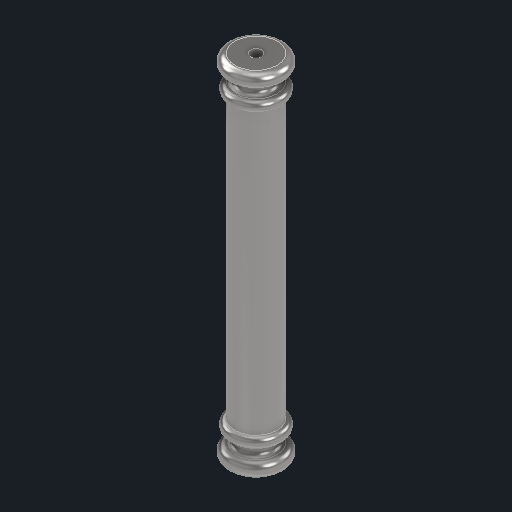
# Autodesk Inventor part: Bell Support Piller
Saved by Autodesk Inventor 2027.1 (Build 311270010, 270A)
## iProperties
Created: 2025-09-17
Material: Stainless Steel
Document SubType Name: Modeling
Designer: SD
Density: 8 g/cm^3
Appearance: Semi-Polished
Mass: 92.5719 g
Surface Area: 49.3716 cm^2
Volume: 11.5715 cm^3
Project: Automatic Tea Steeping mechanism
Part Number: Bell Support Piller
BOM-Mass: 0.09801
BOM-Area: 0.005
DateTimeString: 27-10-25 16:18
Date: 2025-10-27
Length: 100.000 mm
Diameter: 16.000 mm
Procurement: Fabricate - 2nd round
Build Stage: 3
Preferred Material: 303 Stainless Steel
Author: SD
Title: Bell Support Piller
Autodesk Inventor part; units mm, degrees
ref_plane "XZ Plane" through (0, 0, 0) normal (0, 1, 0) x (-1, 0, 0)
ref_plane "XY Plane" through (0, 0, 0) normal (0, 0, 1) x (1, 0, 0)
sketch "Sketch1" plane through (0, 0, 0) normal (0, 0, 1) x (1, 0, 0)
  line L0 (0, 0) -> (0, -100)
  line L1 (0, 0) -> (6, 0)
  line L2 (6, 0) -> (6, -4) construction
  arc A0 (6, -4) -> (6, 0) centre (6, -2) ccw
  arc A1 (6, -4) -> (6, -7) centre (6, -5.5) ccw
  line L3 (6, -5.5) -> (2.7369, -5.5) construction
  arc A2 (6, -10) -> (6, -7) centre (6, -8.5) ccw
  line L4 (0, -100) -> (6, -100)
  line L5 (6, -100) -> (6, -96) construction
  arc A3 (6, -100) -> (6, -96) centre (6, -98) ccw
  arc A4 (6, -93) -> (6, -96) centre (6, -94.5) ccw
  arc A5 (6, -93) -> (6, -90) centre (6, -91.5) ccw
  line L6 (6, -10) -> (6, -90)
  point P0 (6, -90)
  point P1 (6, -10)
  dimension "d1" = 8
  dimension "d2" = 4
  dimension "d3" = 1.5
  dimension "d4" = 3
  dimension "d5" = 3
  dimension "d6" = 1.5
  dimension "d7" = 4
  dimension "d8" = 8
  dimension "d9" = 1.5
  dimension "d10" = 3
  dimension "d11" = 3
  dimension "d12" = 1.5
  dimension "d47" = 80
  constraints: 14 end point, 12 point on circle, 6 centre point, 5 vertical alignment, 4 vertical, 3 horizontal, 2 midpoint
  measures "d2" distance of L1.end L2.end
  measures "d3" radius of A1
  measures "d4" distance of A1.end L2.end
  measures "d5" distance of A1.end L6.start
  measures "d6" radius of A2
  measures "d7" distance of L4.end L5.end
  measures "d9" radius of A4
  measures "d10" distance of L5.end A4.start
  measures "d11" distance of A4.start A5.end
  measures "d12" radius of A5
  measures "d47" distance of L6.start L6.end
revolve "Revolution1" add sketch "Sketch1" angle 360 about axis through (0, 0, 0) along (0, -1, 0)
ref_plane "Work Plane1" through (8, 0, 0) normal (1, 0, 0) x (0, 1, 0)
ref_plane "Work Plane2" through (-8, 0, 0) normal (1, 0, 0) x (0, 1, 0)
sketch "Sketch5" plane through (0, -100, 0) normal (0, -1, 0) x (1, 0, 0)
  point P0 (0, 0)
  point P1 (0, 0)
  constraints: 1 coincident
hole "Hole1" at (0, -100, 0) direction (0, 1, 0) diameter 3.242 depth 20 tip angle 118 thread size "M4x0.7" class "6H" standard "ISO Metric profile"
sketch "Sketch6" plane through (0, 0, 0) normal (0, 1, 0) x (1, 0, 0)
  point P0 (0, 0)
  point P1 (0, 0)
  constraints: 1 coincident
hole "Hole2" at (0, 0, 0) direction (0, -1, 0) diameter 3.242 depth 20 tip angle 118 thread size "M4x0.7" class "6H" standard "ISO Metric profile"
body "Solid1"
